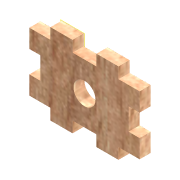
# Autodesk Inventor part: zijkant knoppendoosje met gat
Saved by Autodesk Inventor 2020.3 (Build 243373000, 373)
## iProperties
Created: 2020-12-08
Part Number: zijkant knoppendoosje met gat
Material: Wood (Birch)
Document SubType Name: Sheet Metal
Designer: Svend
Density: 0.55 g/cm^3
Sheet Metal Rule: Default_mm
Appearance: Birch - Natural Polished
Author: Svend
Autodesk Inventor part; units mm, degrees
ref_plane "YZ Plane" through (0, 0, 0) normal (1, 0, 0) x (0, 1, 0)
ref_plane "XZ Plane" through (0, 0, 0) normal (0, 1, 0) x (-1, 0, 0)
ref_plane "XY Plane" through (0, 0, 0) normal (0, 0, 1) x (1, 0, 0)
ref_plane "Work Plane1" through (-25, 0, 0) normal (0, 0, 1) x (1, 0, 0)
sketch "Sketch1" plane through (-25, 0, 0) normal (0, 0, 1) x (1, 0, 0)
  line L0 (25, 6) -> (37, 6)
  line L1 (25, 0) -> (25, 6)
  line L2 (37, 0) -> (25, 0)
  line L3 (37, 0) -> (37, 6)
  line L4 (0, 6) -> (12, 6)
  line L5 (0, 0) -> (0, 6)
  line L6 (12, 0) -> (0, 0)
  line L7 (12, 0) -> (12, 6)
  line L8 (-11.5, 0) -> (0, 0)
  line L9 (12, 0) -> (25, 0)
  line L10 (37, 0) -> (48.5, 0)
  line L11 (48.5, 0) -> (-11.5, 0)
  line L12 (-11.5, -32) -> (48.5, -32)
  line L13 (48.5, -10) -> (42.5, -10)
  line L14 (42.5, -10) -> (42.5, -22)
  line L15 (42.5, -22) -> (48.5, -22)
  line L16 (48.5, -22) -> (48.5, -10)
  line L17 (-11.5, -10) -> (-5.5, -10)
  line L18 (-5.5, -10) -> (-5.5, -22)
  line L19 (-5.5, -22) -> (-11.5, -22)
  line L20 (-11.5, -22) -> (-11.5, -10)
  line L21 (-11.5, 0) -> (-11.5, 6)
  line L22 (48.5, -16) -> (-11.5, -16) construction
  line L23 (25, -38) -> (37, -38)
  line L24 (25, -32) -> (25, -38)
  line L25 (37, -32) -> (25, -32)
  line L26 (37, -32) -> (37, -38)
  line L27 (0, -38) -> (12, -38)
  line L28 (0, -32) -> (0, -38)
  line L29 (12, -32) -> (0, -32)
  line L30 (12, -32) -> (12, -38)
  line L31 (12, -32) -> (25, -32)
  line L32 (48.5, 0) -> (48.5, -32)
  line L33 (-11.5, -32) -> (-11.5, 0)
  point P0 (42.5, -16)
  point P1 (-5.5, -16)
  point P2 (-11.5, -16)
  point P3 (-11.5, -16)
  point P4 (48.5, -16)
  dimension "d0" = 32
  dimension "d1" = 60
  measures "d0" distance of L12.start L11.end
  measures "d1" distance between parallel lines of L32 L33
extrude "Plate1" add sketch "Sketch1" along normal blind 6 contours L0 L3 L2 L1 | L2 L10 L32 L13 L14 L15 L12 L33 L19 L18 L17 L8 L6 L9 | L6 L5 L4 L7 | L26 L23 L24 L12 | L12 L30 L27 L28
sketch "Sketch2" plane through (-25, 0, 6) normal (0, 0, 1) x (1, 0, 0)
  line L0 (-11.5, -10) -> (-5.5, -10) projected
  line L1 (-5.5, -10) -> (-5.5, -22) projected
  line L2 (-5.5, -22) -> (-11.5, -22) projected
  line L3 (-11.5, -32) -> (-11.5, -22) projected
  line L4 (0, -32) -> (-11.5, -32) projected
  line L5 (0, -38) -> (0, -32) projected
  line L6 (12, -38) -> (0, -38) projected
  line L7 (12, -32) -> (12, -38) projected
  line L8 (25, -32) -> (12, -32) projected
  line L9 (25, -38) -> (25, -32) projected
  line L10 (37, -38) -> (25, -38) projected
  line L11 (37, -32) -> (37, -38) projected
  line L12 (48.5, -32) -> (37, -32) projected
  line L13 (48.5, -22) -> (48.5, -32) projected
  line L14 (48.5, -22) -> (42.5, -22) projected
  line L15 (42.5, -22) -> (42.5, -10) projected
  line L16 (42.5, -10) -> (48.5, -10) projected
  line L17 (48.5, 0) -> (48.5, -10) projected
  line L18 (37, 0) -> (48.5, 0) projected
  line L19 (37, 6) -> (37, 0) projected
  line L20 (25, 6) -> (37, 6) projected
  line L21 (25, 0) -> (25, 6) projected
  line L22 (12, 0) -> (25, 0) projected
  line L23 (12, 6) -> (12, 0) projected
  line L24 (0, 6) -> (12, 6) projected
  line L25 (0, 0) -> (0, 6) projected
  line L26 (-11.5, 0) -> (0, 0) projected
  line L27 (-11.5, -10) -> (-11.5, 0) projected
  circle A0 centre (18.5, -16) radius 6
  point P0 (18.5, -32)
  point P1 (42.5, -16)
  dimension "d3" = 12
  constraints: 2 midpoint, 1 centre point, 1 horizontal alignment, 1 vertical alignment
  measures "d3" diameter of A0
extrude "Cut1" cut sketch "Sketch2" against normal blind 6 contours A0
equation "\"d4\" = Thickness"
equation "\"d2\" = Thickness"
equation "\"BendRadius\" = Thickness"
equation "\"BendReliefWidth\" = Thickness"
equation "\"BendReliefDepth\" = 0.5 * Thickness"
equation "\"CornerReliefSize\" = 4 * Thickness"
equation "\"MinimumRemnant\" = 2 * Thickness"
equation "\"TransitionRadius\" = BendRadius"
equation "\"JacobiRadiusSize\" = BendRadius"
equation "\"GapSize\" = Thickness"
equation "\"Thickness\" = 6"
body "Solid1"
